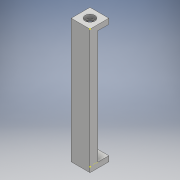
# Autodesk Inventor part: baseAxel 11-28
Saved by Autodesk Inventor 2018 (Build 220112000, 112)
## iProperties
Created: 2019-11-28
Part Number: baseAxel 11-28
Material: Generic
Document SubType Name: Modeling
Designer: Aditya Kendre
Density: 1 g/cm^3
Appearance: Default
Author: Aditya Kendre
Autodesk Inventor part; units mm, degrees
ref_plane "YZ Plane" through (0, 0, 0) normal (1, 0, 0) x (0, 1, 0)
ref_plane "XZ Plane" through (0, 0, 0) normal (0, 1, 0) x (-1, 0, 0)
ref_plane "XY Plane" through (0, 0, 0) normal (0, 0, 1) x (1, 0, 0)
sketch "Sketch1" plane through (0, 0, 0) normal (0, 1, 0) x (-1, 0, 0)
  line L0 (0, 0) -> (25, 0)
  line L1 (25, 0) -> (25, -165)
  line L2 (25, -165) -> (0, -165)
  line L3 (0, -165) -> (0, 0)
  dimension "d0" = 25
  dimension "d1" = 165
  constraints: 8 end point, 2 parallel, 1 horizontal, 1 perpendicular
  measures "d0" distance of L1.end L2.end
  measures "d1" distance of L0.end L1.end
extrude "Extrusion1" add sketch "Sketch1" along normal blind 3
sketch "Sketch2" plane through (0, 3, 0) normal (0, 1, 0) x (1, 0, 0)
  line L0 (-25, 165) -> (-25, 0) projected
  line L1 (0, 0) -> (0, 165) projected
  line L2 (-25, 0) -> (0, 0)
  line L3 (0, 0) -> (0, 7)
  line L4 (0, 7) -> (-25, 7)
  line L5 (-25, 7) -> (-25, 0)
  line L6 (0, 165) -> (-25, 165) projected
  line L7 (-25, 165) -> (0, 165)
  line L8 (0, 165) -> (0, 158)
  line L9 (0, 158) -> (-25, 158)
  line L10 (-25, 158) -> (-25, 165)
  dimension "d4" = 7
  dimension "d5" = 7
  constraints: 16 end point, 4 parallel, 2 horizontal, 2 perpendicular, 2 point on line
  measures "d4" distance of L3.end L2.end
  measures "d5" distance of L7.end L8.end
extrude "Extrusion2" add sketch "Sketch2" along normal blind 22 contours L6 L1 L9 L0 | L4 L1 L2 L0
sketch "Sketch3" plane through (-25, 0, 0) normal (0, 0, 1) x (1, 0, 0)
  point P0 (25, 0)
sketch "Sketch4" plane through (-25, 0, 0) normal (0, 0, 1) x (1, 0, 0)
  line L0 (25, 25) -> (0, 25) construction
  line L1 (25, 0) -> (0, 25) construction
  circle A0 centre (12.5, 12.5) radius 6.5
  dimension "d8" = 13
  constraints: 2 end point, 1 centre point, 1 coincident, 1 midpoint
  measures "d8" diameter of A0
extrude "Extrusion3" cut sketch "Sketch4" against normal blind 5
sketch "Sketch5" plane through (0, 0, -165) normal (0, 0, -1) x (-1, 0, 0)
  circle A0 centre (12.5, 12.5) radius 6.5 projected
  circle A1 centre (12.5, 12.5) radius 6.5
  point P0 (0, 0)
  constraints: 1 centre point, 1 coincident
extrude "Extrusion4" cut sketch "Sketch5" against normal blind 5
sketch "Sketch6" plane through (-25, 0, 0) normal (0, 0, 1) x (1, 0, 0)
  circle A0 centre (12.5, 12.5) radius 6.5 projected
  circle A1 centre (12.5, 12.5) radius 5
  point P0 (25, 0)
  dimension "d13" = 10
  constraints: 1 centre point, 1 coincident
  measures "d13" diameter of A1
extrude "Extrusion5" cut sketch "Sketch6" against normal blind 165 contours A1
sketch "Sketch7" plane through (-25, 3, -158) normal (0, 0, 1) x (1, 0, 0)
  line L0 (25, 0) -> (25, 22) construction
  line L1 (0, 0) -> (0, 22) construction
  point P0 (25, -3)
sketch "Sketch8" plane through (-25, 3, -158) normal (0, 0, 1) x (1, 0, 0)
  circle A0 centre (12.5, 9.5) radius 5 projected
  point P0 (25, -3)
  constraints: 1 coincident
sketch "Sketch9" plane through (0, 3, 0) normal (0, 1, 0) x (1, 0, 0)
  line L0 (-25, 158) -> (0, 158) projected
  line L1 (0, 7) -> (-25, 7) projected
  line L2 (-25, 158) -> (-20, 158)
  line L3 (-20, 158) -> (-20, 7)
  line L4 (-20, 7) -> (-25, 7)
  line L5 (-25, 7) -> (-25, 158)
  line L6 (0, 0) -> (0, 7) projected
  line L7 (0, 7) -> (-5, 7)
  line L8 (-5, 7) -> (-5, 158)
  line L9 (-5, 158) -> (0, 158)
  line L10 (0, 158) -> (0, 7)
  dimension "d16" = 5
  dimension "d17" = 5
  constraints: 16 end point, 4 parallel, 2 horizontal, 2 perpendicular, 2 point on line
  measures "d16" distance of L3.end L4.end
  measures "d17" distance of L8.end L9.end
extrude "Extrusion6" add sketch "Sketch9" along normal blind 7.5 contours L0 L3 L1 L5 | L0 L10 L1 L8
fillet "Fillet1" radius 2 2 edges at (-5, 10.5, -82.5) (-20, 10.5, -82.5)
body "Solid1"
